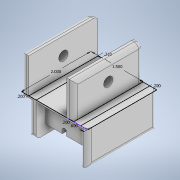
# Autodesk Inventor part: Sample Holder end for 8020-forelveflowmbd
Saved by Autodesk Inventor 2020 (Build 240168000, 168)
## iProperties
Created: 2022-02-15
Part Number: Sample Holder end for 8020-forelveflowmbd
Material: Generic
Document SubType Name: Modeling
Designer: Beaucage
Density: 1 g/cm^3
Appearance: Default
Author: Beaucage
Autodesk Inventor part; units mm, degrees
ref_plane "YZ Plane" through (0, 0, 0) normal (1, 0, 0) x (0, 1, 0)
ref_plane "XZ Plane" through (0, 0, 0) normal (0, 1, 0) x (-1, 0, 0)
ref_plane "XY Plane" through (0, 0, 0) normal (0, 0, 1) x (1, 0, 0)
sketch "Sketch1" plane through (0, 0, 0) normal (0, 1, 0) x (-1, 0, 0)
  line L0 (0, 0) -> (38.1, 0)
  line L1 (38.1, 0) -> (38.1, -50.8)
  line L2 (38.1, -50.8) -> (0, -50.8)
  line L3 (0, -50.8) -> (0, 0)
  line L4 (38.1, -50.8) -> (33.02, -50.8)
  line L5 (33.02, -50.8) -> (33.02, 0)
  line L6 (33.02, 0) -> (38.1, 0)
  line L7 (38.1, 0) -> (38.1, -50.8)
  line L8 (0, -50.8) -> (5.08, -50.8)
  line L9 (5.08, -50.8) -> (5.08, 0)
  line L10 (5.08, 0) -> (0, 0)
  line L11 (0, 0) -> (0, -50.8)
  line L12 (5.08, -50.8) -> (-10.16, -50.8)
  line L13 (-10.16, -50.8) -> (-10.16, 0)
  line L14 (-10.16, 0) -> (5.08, 0)
  line L15 (5.08, 0) -> (5.08, -50.8)
  line L16 (-10.16, 0) -> (-5.08, 0)
  line L17 (-5.08, 0) -> (-5.08, -50.8)
  line L18 (-5.08, -50.8) -> (-10.16, -50.8)
  line L19 (-10.16, -50.8) -> (-10.16, 0)
  line L20 (33.02, -50.8) -> (27.686, -50.8)
  line L21 (27.686, -50.8) -> (27.686, 0)
  line L22 (33.02, 0) -> (27.686, 0)
  dimension "d0" = 38.1
  dimension "d1" = 50.8
  dimension "d2" = 5.08
  dimension "d3" = 5.08
  dimension "d16" = 15.24
  dimension "d17" = 5.08
  dimension "d37" = 5.334
  constraints: 46 end point, 10 parallel, 6 perpendicular, 5 horizontal, 5 point on line, 1 collinear
  measures "d0" distance of L1.end L2.end
  measures "d1" distance of L0.end L1.end
  measures "d2" distance of L5.end L6.end
  measures "d3" distance of L10.end L9.end
  measures "d16" distance of L13.end L14.end
  measures "d17" distance of L17.end L18.end
  measures "d37" distance of L4.end L20.end
extrude "Extrusion1" add sketch "Sketch1" along normal blind 25.4 contours L0 L9 L2 L3 | L0 L1 L2 L5
extrude "Extrusion2" add sketch "Sketch1" against normal blind 1.27
sketch "Sketch2" plane through (0, 25.4, 0) normal (1, 0, 0) x (0, 0, -1)
  line L0 (50.8, 0) -> (0, 0) projected
  line L1 (25.4, 0) -> (25.4, -12.7)
  point P0 (0, -25.4)
  dimension "d8" = 12.7
  constraints: 2 end point, 1 midpoint, 1 vertical
  measures "d8" distance of L1.start L1.end
hole "Hole1" at (0, 12.7, -25.4) direction (-1, 0, 0) diameter 6.7564 end through all clearance for "Socket Head Cap Screw" size "1/4" standard "Ansi Unified Screw Threads"
extrude "Extrusion3" add sketch "Sketch1" against normal blind 25.4 contours L17 L12 L13 L14 | L0 L5 L2 L21
sketch "Sketch3" plane through (0, -1.27, 0) normal (0, -1, 0) x (1, 0, 0)
  line L0 (10.16, -50.8) -> (10.16, 0) projected
  line L1 (10.16, -25.4) -> (10.16, -10.4)
  line L2 (10.16, -10.4) -> (10.16, -40.4)
  line L3 (-38.1, -50.8) -> (-38.1, 0) projected
  line L4 (10.16, -10.4) -> (-38.1, -10.4)
  line L5 (-38.1, -10.4) -> (-38.1, -7.225)
  line L6 (-38.1, -7.225) -> (10.16, -7.225)
  line L7 (10.16, -7.225) -> (10.16, -10.4)
  line L8 (10.16, -40.4) -> (-38.1, -40.4)
  line L9 (-38.1, -40.4) -> (-38.1, -43.575)
  line L10 (-38.1, -43.575) -> (10.16, -43.575)
  line L11 (10.16, -43.575) -> (10.16, -40.4)
  point P0 (0, 0)
  point P1 (10.16, -43.575)
  point P2 (-38.1, -40.4)
  point P3 (10.16, -7.225)
  point P4 (-38.1, -10.4)
  dimension "d23" = 15
  dimension "d24" = 30
  dimension "d25" = 3.175
  dimension "d26" = 3.175
  constraints: 20 end point, 4 parallel, 4 point on line, 2 horizontal, 2 perpendicular, 1 midpoint
  measures "d23" distance of L1.start L1.end
  measures "d24" distance of L1.end L2.end
  measures "d25" distance of L4.end L5.end
  measures "d26" distance of L9.end L8.end
extrude "Extrusion4" add sketch "Sketch3" along normal blind 17.78 contours L10 L3 L8 L0 | L4 L3 L6 L0
sketch "Sketch4" plane through (5.08, -1.27, -43.575) normal (0, 0, -1) x (-1, 0, 0)
  line L0 (38.1, 0) -> (38.1, -24.13) projected
  line L1 (38.1, -17.7558) -> (19.05, -17.7558)
  line L2 (0, -17.78) -> (32.766, -17.78) projected
  line L3 (38.1, -17.7558) -> (57.15, -17.7558) construction
  line L4 (19.05, -20.2958) -> (19.05, -15.2158) construction
  line L5 (20.6375, -20.2958) -> (20.6375, -15.2158)
  line L6 (17.4625, -15.2158) -> (17.4625, -20.2958)
  arc A0 (17.4625, -20.2958) -> (20.6375, -20.2958) centre (19.05, -20.2958) ccw
  arc A1 (20.6375, -15.2158) -> (17.4625, -15.2158) centre (19.05, -15.2158) ccw
  point P0 (5.08, 1.27)
  point P1 (38.1, -17.78)
  point P2 (17.4625, -17.78)
  point P3 (20.6375, -17.78)
  dimension "d29" = 19.05
  dimension "d30" = 180
  dimension "d31" = 2.54
  dimension "d32" = 3.175
  constraints: 12 end point, 4 point on circle, 4 tangent, 2 centre point, 2 parallel, 1 collinear, 1 horizontal, 1 midpoint, 1 point on line, 1 vertical
  measures "d29" distance of L1.start L1.end
  measures "d30" angle of L1 L3
  measures "d31" distance of L1.end L4.end
  measures "d32" diameter of A1
extrude "Extrusion5" cut sketch "Sketch4" against normal through all contours L6 A1 L5 L2
fillet "Fillet1" radius 3.175 9 edges at (-38.1, 12.065, -50.8) (0, 12.7, -50.8) (10.16, -12.7, -50.8) (10.16, -25.4, -25.4) (10.16, -12.7, 0) (-35.56, -1.27, -43.575) (-11.303, -1.27, -43.575) (-33.02, -10.16, -43.575) (5.08, -10.16, -43.575)
fillet "Fillet2" radius 3.175 15 edges at (-35.56, -1.27, -7.225) (-11.303, -1.27, -7.225) (-33.02, -10.16, -7.225) (-33.02, -13.335, 0) (5.08, -13.335, 0) (0, 12.7, 0) (-0.9299, 25.4, -49.8701) (-4.1275, 25.4, -50.8) (0, 25.4, -23.8125) (-30.353, -25.4, 0) (-38.1, 12.065, 0) (5.08, -10.16, -7.225) (-37.1701, 25.4, -49.8701) (-33.9725, 25.4, -50.8) (-38.1, 25.4, -23.8125)
body "Solid1"
